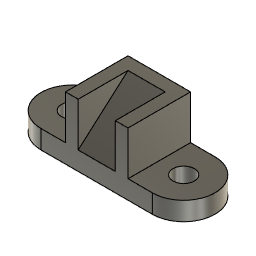
A2 (Autodesk Fusion 360 design; units mm, degrees)
Autodesk Fusion 360 part; units mm, degrees
sketch "Sketch1" plane through (0, 0, 0) normal (0, 0, 1) x (1, 0, 0)
  line L0 (57, 32) -> (-57, 32)
  line L1 (-57, 32) -> (-57, -32)
  line L2 (-57, -32) -> (57, -32)
  line L3 (57, -32) -> (57, 32)
  line L4 (57, 32) -> (-57, -32) construction
  line L5 (-57, 32) -> (57, -32) construction
  line L6 (32, -32) -> (32, 32)
  line L7 (19, -32) -> (19, 19)
  line L8 (19, 19) -> (-19, 19)
  line L9 (-19, 19) -> (-19, -32)
  line L10 (-32, -32) -> (-32, 32)
  line L11 (0, 32) -> (0, -32) construction
  circle A0 centre (57, 0) radius 11
  circle A1 centre (-57, 0) radius 11
  circle A2 centre (57, 0) radius 32
  circle A3 centre (-57, 0) radius 32
  dimension "d1" = 114
  dimension "d2" = 64
  dimension "d3" = 51
  dimension "d4" = 38
  dimension "d5" = 64
  dimension "d6" = 22
  dimension "d7" = 22
  dimension "d8" = 64
  dimension "d9" = 64
  constraint horizontal L0
  constraint perpendicular L0 L1
  constraint parallel L0 L2
  constraint parallel L1 L3
  constraint coincident L4 origin
  constraint coincident L5 origin
  constraint coincident L2 L6.start
  constraint coincident L0 L6.end
  constraint perpendicular L0 L6
  constraint coincident L2 L7.start
  constraint perpendicular L2 L7
  constraint perpendicular L7 L8
  constraint coincident L2 L9.end
  constraint perpendicular L2 L9
  constraint coincident L2 L10.start
  constraint coincident L0 L10.end
  constraint perpendicular L0 L10
  constraint midpoint L0 L11.start
  constraint midpoint L2 L11.end
  constraint symmetric L7 L9 L11
  constraint symmetric L6 L10 L11
  constraint midpoint L3 A0.centre
  constraint concentric A0 A2
  measures "d1" distance of L1.end L2.end
  measures "d2" distance of L0.end L1.end
  measures "d3" distance of L7.start L7.end
  measures "d4" distance of L7.end L8.end
  measures "d5" distance of L6.end L10.end
  measures "d6" diameter of A0
  measures "d7" diameter of A1
  measures "d8" diameter of A2
  measures "d9" diameter of A3
extrude "Extrude2" add sketch "Sketch1" along normal blind 19 contours L1 A1 A3 makes body 1
extrude "Extrude1" add sketch "Sketch1" along normal blind 19 separate body contours L3 A0 A2 makes body 2
extrude "Extrude3" add sketch "Sketch1" along normal blind 19 contours L1 L10 A1 A3 bodies 1
extrude "Extrude4" add sketch "Sketch1" along normal blind 19 contours L0 L6 A2 | L3 L6 A0 A2 | L0 L10 A3 | L2 L6 A2 | L2 L10 A3 bodies 1 2
extrude "Extrude5" add sketch "Sketch1" along normal blind 64 contours L0 L2 L6 L7 L8 L9 L10 A2 A3 | L6 A2 | L10 A3 bodies 1 2
ref_plane "WorkPlane1" through (0, -6.5, 32) normal (-1, 0, 0) x (0, -1, 0)
sketch "Sketch2" plane through (0, -6.5, 32) normal (-1, 0, 0) x (0, 1, 0)
extrude "Extrude6" add sketch "Sketch1" along normal blind 19 contours L2 L7 L8 L9 bodies 1
ref_plane "WorkPlane2" through (0, -6.5, 41.5) normal (1, 0, 0) x (0, 1, 0)
sketch "Sketch4" plane through (0, 19, 0) normal (0, -1, 0) x (1, 0, 0)
  line L0 (-19, 19) -> (19, 19)
  line L1 (19, 19) -> (19, 64)
  line L2 (19, 64) -> (-19, 64)
  line L3 (-19, 64) -> (-19, 19)
  line L4 (0, 64) -> (0, 19) construction
  constraint midpoint L2 L4.start
  constraint midpoint L0 L4.end
sketch "Sketch5" plane through (0, 19, 0) normal (0, -1, 0) x (1, 0, 0)
sketch "Sketch6" plane through (0, 0, 19) normal (0, 0, 1) x (-1, 0, 0)
  line L0 (19, -19) -> (19, 32)
  line L1 (19, 32) -> (-19, 32)
  line L2 (-19, 32) -> (-19, -19)
  line L3 (-19, -19) -> (19, -19)
  line L4 (0, -19) -> (0, 32) construction
  constraint midpoint L3 L4.start
  constraint midpoint L1 L4.end
sketch "Sketch3" plane through (0, -6.5, 41.5) normal (1, 0, 0) x (0, 1, 0)
  line L0 (25.5, 22.5) -> (-25.5, -22.5)
  line L1 (-25.5, -22.5) -> (25.5, -22.5)
  line L2 (25.5, -22.5) -> (25.5, 22.5)
  point P0 (6.5, -22.5)
  point P1 (-25.5, -22.5)
  point P2 (25.5, -22.5)
  point P3 (25.5, 22.5)
  constraint horizontal L1
  constraint vertical L2
  constraint coincident L1 P0
  constraint coincident P1 L0.end
  constraint coincident P2 L1.end
  constraint coincident P3 L0.start
extrude "Extrude7" add sketch "Sketch3" along normal up to surface (-19 mm away) and the other way up to surface (-19 mm away) bodies 1
